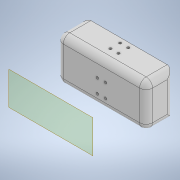
# Autodesk Inventor part: Soporte_Brazo_dcho
Saved by Autodesk Inventor 2021 (Build 250183000, 183)
## iProperties
Created: 2022-01-19
Part Number: Soporte_Brazo_dcho
Material: Genérico
Document SubType Name: Modeling
Designer: Joaquín
Density: 1 g/cm^3
Appearance: Valor por defecto
Author: Joaquín
Autodesk Inventor part; units mm, degrees
ref_plane "YZ Plane" through (0, 0, 0) normal (1, 0, 0) x (0, 1, 0)
ref_plane "XZ Plane" through (0, 0, 0) normal (0, 1, 0) x (-1, 0, 0)
ref_plane "XY Plane" through (0, 0, 0) normal (0, 0, 1) x (1, 0, 0)
sketch "Boceto1" plane through (0, 0, 0) normal (0, 1, 0) x (-1, 0, 0)
  line L0 (0, 0) -> (0, -24)
  line L1 (10, 0) -> (0, 0)
  line L2 (55, -24) -> (55, 0)
  line L3 (55, 0) -> (10, 0)
  line L4 (0, -24) -> (0, -34)
  line L5 (0, -34) -> (55, -34)
  line L6 (55, -34) -> (55, -24)
  line L7 (0, 0) -> (5, 0)
  circle A0 centre (5, -6) radius 1.5
  circle A1 centre (5, -18) radius 1.5
  dimension "d0" = 24
  dimension "d4" = 10
  dimension "d7" = 5
  constraints: 16 end point, 2 centre point, 2 vertical, 1 collinear, 1 midpoint, 1 perpendicular
  measures "d0" distance of L0.start L0.end
  measures "d4" distance of L0.end L4.end
  measures "d7" distance of L0.start L7.end
extrude "Extrusión1" add sketch "Boceto1" along normal blind 8
sketch "Boceto2" plane through (0, 0, 0) normal (0, -1, 0) x (1, 0, 0)
  line L0 (0, 0) -> (0, -24.5)
  line L1 (0, 0) -> (0, -34) projected
  line L2 (0, -24.5) -> (-46, -24.5)
  line L3 (-55, -34) -> (-55, 0) projected
  line L4 (-55, -24.5) -> (-55, -34)
  line L5 (0, -34) -> (-55, -34) projected
  line L6 (0, -34) -> (-55, -34)
  line L7 (0, -34) -> (0, -24.5)
  line L8 (-55, 0) -> (0, 0) projected
  line L9 (-55, 0) -> (-46, 0)
  line L10 (-46, 0) -> (-46, -24.5)
  line L11 (-55, -24.5) -> (-55, 0)
  dimension "d15" = 24.5
  dimension "d16" = 9
  constraints: 16 end point, 4 collinear, 3 point on line, 2 perpendicular
  measures "d15" distance of L0.start L0.end
  measures "d16" distance of L3.end L9.end
extrude "Extrusión2" add sketch "Boceto2" along normal blind 45 contours L1 L5 L3 L8 L10 L2
sketch "Boceto3" plane through (0, 8, -34) normal (0, 0, -1) x (-1, 0, 0)
  circle A0 centre (5, -23) radius 1.5
  circle A1 centre (5, -40) radius 1.5
  point P0 (0, -8)
  constraints: 2 centre point
extrude "Extrusión3" cut sketch "Boceto3" against normal blind 45
fillet "Empalme1" radius 8 6 edges at (-27.5, 8, -34) (-55, -18.5, -34) (-55, 8, -17) (-27.5, -45, -34) (-55, -18.5, 0) (-55, -45, -17)
mirror "Simetría1" about plane through (0, 0, 0) normal (1, 0, 0)
ref_plane "Plano de trabajo3" through (-47, -37, -96.25) normal (0, 0, -1) x (-1, 0, 0)
mirror "Simetría3" about plane through (-47, -37, -96.25) normal (0, 0, -1) remove original yes
